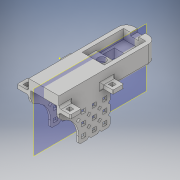
# Autodesk Inventor part: Milling Machine with light_sensor_mount
Saved by Autodesk Inventor 2017 SP1 (Build 210196100, 196)
## iProperties
Created: 2016-11-04
Part Number: Milling Machine with light_sensor_mount
Material: Generic
Document SubType Name: Modeling
Designer: rmainhar
Density: 1 g/cm^3
Appearance: Default
Author: rmainhar
Autodesk Inventor part; units mm, degrees
ref_plane "YZ Plane" through (0, 0, 0) normal (1, 0, 0) x (0, 1, 0)
ref_plane "XZ Plane" through (0, 0, 0) normal (0, 1, 0) x (-1, 0, 0)
ref_plane "XY Plane" through (0, 0, 0) normal (0, 0, 1) x (1, 0, 0)
sketch "Sketch1" plane through (0, 0, 0) normal (0, 1, 0) x (-1, 0, 0)
  line L0 (0, -12.7) -> (-63.5, -12.7)
  line L1 (-63.5, -12.7) -> (-63.5, 0)
  line L2 (-63.5, 0) -> (0, 0)
  line L3 (0, 0) -> (0, -12.7)
  line L4 (-3.9687, -7.9375) -> (-8.7313, -7.9375)
  line L5 (-8.7313, -7.9375) -> (-8.7312, -3.175)
  line L6 (-8.7312, -3.175) -> (-3.9687, -3.175)
  line L7 (-3.9687, -3.175) -> (-3.9687, -7.9375)
  line L8 (-54.7687, -3.175) -> (-54.7687, -7.9375)
  line L9 (-54.7687, -7.9375) -> (-59.5312, -7.9375)
  line L10 (-59.5312, -3.175) -> (-54.7687, -3.175)
  line L11 (-59.5312, -7.9375) -> (-59.5312, -3.175)
  point P0 (0, 0)
  dimension "d0" = 63.5
  dimension "d1" = 4.7625
  dimension "d2" = 4.7625
  dimension "d4" = 3.175
  dimension "d5" = 12.7
  dimension "d6" = 3.9688
  dimension "d9" = 50.8
  dimension "d14" = 3.9688
  constraints: 24 end point, 4 parallel, 3 horizontal, 2 perpendicular, 1 coincident, 8 other
  measures "d0" distance of L1.end L2.end
  measures "d1" distance of L5.end L6.end
  measures "d2" distance of L4.end L5.end
  measures "d4" distance between parallel lines of L2 L6
  measures "d5" distance of L2.end L0.start
  measures "d6" distance between parallel lines of L3 L7
  measures "d9" distance of L6.end L8.start
  measures "d14" distance between parallel lines of L1 L11
extrude "Extrusion1" add sketch "Sketch1" along normal blind 3.175
sketch "Sketch2" plane through (0, 0, 0) normal (0, -1, 0) x (1, 0, 0)
  line L0 (41.91, -43.3549) -> (21.8148, -43.3549)
  line L1 (21.8148, -43.3549) -> (21.8148, -12.7)
  line L2 (21.8148, -12.7) -> (41.91, -12.7)
  line L3 (41.91, -12.7) -> (41.91, -43.3549)
  line L4 (0, -12.7) -> (63.5, -12.7) projected
  line L5 (63.5, -12.7) -> (0, -12.7) projected
  line L6 (31.75, -12.7) -> (31.75, 0)
  line L7 (48.26, -49.7049) -> (15.4648, -49.7049)
  line L8 (15.4648, -49.7049) -> (15.4648, -6.35)
  line L9 (15.4648, -6.35) -> (48.26, -6.35)
  line L10 (48.26, -6.35) -> (48.26, -49.7049)
  point P0 (0, 0)
  dimension "d17" = 20.32
  dimension "d18" = 6.35
  dimension "d81" = 30.6549
  constraints: 18 end point, 4 parallel, 2 perpendicular, 1 horizontal, 1 midpoint, 1 point on line, 1 vertical, 3 other
  measures "d17" diameter of L3 L6
  measures "d18" distance between parallel lines of L10 L3
  measures "d81" distance between parallel lines of L0 L4
extrude "Extrusion2" add sketch "Sketch2" along normal blind 10.16 contours L3 L4 L10 L7 L8 L1 L0 | L2 L6 L9 L10 L4 | L4 L8 L9 L6 L2
sketch "Sketch3" plane through (63.5, 3.175, -12.7) normal (0, 0, -1) x (-1, 0, 0)
  line L0 (21.59, -13.335) -> (41.6852, -13.335) projected
  line L1 (41.6852, -13.335) -> (21.59, -13.335) projected
  line L2 (48.0352, -13.335) -> (15.24, -13.335) projected
  line L3 (15.24, -13.335) -> (48.0352, -13.335) projected
  line L4 (63.5, -3.175) -> (48.0352, -3.175) projected
  line L5 (63.5, -3.175) -> (63.5, 0) projected
  line L6 (0, 0) -> (63.5, 0) projected
  line L7 (0, -3.175) -> (0, 0) projected
  line L8 (15.24, -3.175) -> (0, -3.175) projected
  line L9 (21.59, -3.175) -> (15.24, -3.175) projected
  line L10 (21.59, -3.175) -> (21.59, -13.335) projected
  line L11 (41.6852, -13.335) -> (21.59, -13.335) projected
  line L12 (41.6852, -3.175) -> (41.6852, -13.335) projected
  line L13 (48.0352, -3.175) -> (41.6852, -3.175) projected
  line L14 (21.59, -3.175) -> (41.6852, -3.175)
  line L15 (41.6852, -3.175) -> (41.6852, -13.335)
  line L16 (41.6852, -13.335) -> (21.59, -13.335)
  line L17 (21.59, -13.335) -> (21.59, -3.175)
  constraints: 8 end point, 2 parallel, 1 horizontal, 1 perpendicular
extrude "Extrusion3" cut sketch "Sketch3" against normal blind 12.7 contours L10 L14 L12 L0
sketch "Sketch4" plane through (0, 0, 0) normal (0, 1, 0) x (1, 0, 0)
  line L0 (41.91, 12.7) -> (48.26, 12.7) projected
  line L1 (48.26, 12.7) -> (48.26, 49.7049) projected
  line L2 (48.26, 49.7049) -> (15.4648, 49.7049) projected
  line L3 (15.4648, 49.7049) -> (15.4648, 12.7) projected
  line L4 (21.8148, 12.7) -> (21.8148, 43.3549) projected
  line L5 (21.8148, 43.3549) -> (41.91, 43.3549) projected
  line L6 (41.91, 43.3549) -> (41.91, 12.7) projected
  line L7 (15.4648, 12.7) -> (21.8148, 12.7) projected
  point P0 (0, 0)
extrude "Extrusion4" add sketch "Sketch4" along normal up to surface (3.175 mm away)
sketch "Sketch5" plane through (41.91, 0, -12.7) normal (0, 0, -1) x (-1, 0, 0)
  line L0 (0, 3.175) -> (0, 0) projected
  line L1 (0, 0) -> (20.0952, 0) projected
  line L2 (20.0952, 0) -> (20.0952, 3.175) projected
  line L3 (0, 3.175) -> (20.0952, 3.175) projected
  point P0 (41.91, 0)
extrude "Extrusion5" cut sketch "Sketch5" against normal through all
sketch "Sketch6" plane through (41.91, 0, -6.35) normal (-1, 0, 0) x (0, 0, 1)
  line L0 (0, 0) -> (-6.35, 0) projected
  line L1 (0, 0) -> (0, -10.16) projected
  line L2 (-43.3549, -10.16) -> (0, -10.16) projected
  line L3 (-43.3549, 3.175) -> (-43.3549, -10.16) projected
  line L4 (-43.3549, 3.175) -> (-6.35, 3.175) projected
  line L5 (-6.35, 0) -> (-6.35, 3.175) projected
  line L6 (3.175, 0) -> (3.175, 3.175) projected
  line L7 (-6.35, 0) -> (6.35, 0) projected
  line L8 (-6.35, 0) -> (-6.35, 3.175) projected
  line L9 (6.35, 3.175) -> (-6.35, 3.175) projected
  line L10 (6.35, 0) -> (6.35, 3.175) projected
  line L11 (-43.3549, -10.16) -> (0, -10.16) projected
  arc A0 (0, -10.16) -> (6.35, 0) centre (-4.953, 0) ccw
  line L12 (0, 0) -> (0, -10.16) projected
  line L13 (0, -10.16) -> (0, 0)
  line L14 (6.35, 0) -> (0, 0) projected
  line L15 (0, 0) -> (6.35, 0)
  constraints: 4 end point, 2 point on circle, 1 centre point, 1 collinear, 1 perpendicular, 1 tangent
extrude "Extrusion6" add sketch "Sketch6" against normal up to surface (6.35 mm away) contours L7 A0 L1
sketch "Sketch17" plane through (0, 0, 0) normal (0, -1, 0) x (1, 0, 0)
  line L0 (21.8148, -6.35) -> (21.8148, 0) projected
  line L1 (21.8148, 0) -> (0, 0) projected
  line L2 (0, 0) -> (0, -12.7) projected
  line L3 (0, -12.7) -> (15.4648, -12.7) projected
  line L4 (15.4648, -12.7) -> (15.4648, -6.35) projected
  line L5 (15.4648, -6.35) -> (21.8148, -6.35) projected
  line L6 (8.7312, -3.175) -> (8.7313, -7.9375) projected
  line L7 (8.7313, -7.9375) -> (3.9687, -7.9375) projected
  line L8 (3.9687, -7.9375) -> (3.9687, -3.175) projected
  line L9 (3.9687, -3.175) -> (8.7312, -3.175) projected
  point P0 (0, 0)
sketch "Sketch7" plane through (0, -10.16, 0) normal (0, -1, 0) x (1, 0, 0)
  line L0 (48.26, 0) -> (48.26, -12.7) projected
  line L1 (48.26, -12.7) -> (63.5, -12.7) projected
  line L2 (63.5, -12.7) -> (63.5, 0) projected
  line L3 (63.5, 0) -> (48.26, 0) projected
  line L4 (54.7687, -7.9375) -> (54.7687, -3.175) projected
  line L5 (54.7687, -3.175) -> (59.5312, -3.175) projected
  line L6 (59.5312, -3.175) -> (59.5312, -7.9375) projected
  line L7 (59.5312, -7.9375) -> (54.7687, -7.9375) projected
  line L8 (41.91, -6.35) -> (41.91, -43.3549) projected
  line L9 (41.91, -43.3549) -> (21.8148, -43.3549) projected
  line L10 (21.8148, -43.3549) -> (21.8148, -6.35) projected
  line L11 (21.8148, -6.35) -> (15.4648, -6.35) projected
  line L12 (15.4648, -6.35) -> (15.4648, -49.7049) projected
  line L13 (15.4648, -49.7049) -> (48.26, -49.7049) projected
  line L14 (48.26, -49.7049) -> (48.26, -6.35) projected
  line L15 (48.26, -6.35) -> (41.91, -6.35) projected
  line L16 (41.91, -43.3549) -> (41.91, 0) projected
  line L17 (41.91, 0) -> (63.5, 0) projected
  line L18 (48.26, 0) -> (41.91, 0)
  line L19 (41.91, 0) -> (41.91, -12.7)
  arc A0 (46.814, 0) -> (41.91, -12.7) centre (60.8067, -12.7) ccw
  line L20 (41.91, -6.35) -> (41.91, -43.3549) projected
  point P0 (0, 0)
  constraints: 4 end point, 2 point on circle, 2 point on line, 1 centre point, 1 collinear, 1 perpendicular, 1 tangent
extrude "Extrusion8" cut sketch "Sketch7" against normal through all contours A0 L15 L16 L17 | A0 L8 L15
ref_plane "Work Plane1" through (31.8624, -10.16, -43.3549) normal (-1, 0, 0) x (0, 0, 1)
mirror "Mirror1" about plane through (31.8624, -10.16, -43.3549) normal (-1, 0, 0) of "Extrusion8", "Extrusion6"
fillet "Fillet10" radius 1.524 5 edges at (42.1867, -10.16, -9.4778) (41.91, -10.16, -28.0275) (21.5381, -10.16, -9.4778) (21.8148, -10.16, -28.0275) (31.8624, -10.16, -43.3549)
sketch "Sketch8" plane through (0, 3.175, 0) normal (0, 1, 0) x (1, 0, 0)
  point P0 (0, 0)
sketch "Sketch9" plane through (0, 3.175, 0) normal (0, 1, 0) x (1, 0, 0)
  line L0 (13.8138, 65.5799) -> (49.911, 65.5799)
  line L1 (49.911, 65.5799) -> (49.911, -57.15)
  line L2 (49.911, -57.15) -> (13.8138, -57.15)
  line L3 (13.8138, -57.15) -> (13.8138, 65.5799)
  line L4 (15.4648, 49.7049) -> (48.26, 49.7049) projected
  line L5 (15.4648, 12.7) -> (15.4648, 49.7049) projected
  line L6 (15.4648, 12.7) -> (0, 12.7) projected
  line L7 (0, 12.7) -> (0, 0) projected
  line L8 (0, 0) -> (16.9108, 0) projected
  arc A0 (16.9108, 0) -> (21.8148, 12.7) centre (2.9181, 12.7) ccw projected
  line L9 (21.8148, 43.3549) -> (21.8148, 12.7) projected
  line L10 (41.91, 43.3549) -> (21.8148, 43.3549) projected
  line L11 (41.91, 43.3549) -> (41.91, 12.7) projected
  arc A1 (41.91, 12.7) -> (46.814, 0) centre (60.8067, 12.7) ccw projected
  line L12 (46.814, 0) -> (63.5, 0) projected
  line L13 (63.5, 0) -> (63.5, 12.7) projected
  line L14 (63.5, 12.7) -> (48.26, 12.7) projected
  line L15 (48.26, 49.7049) -> (48.26, 12.7) projected
  line L16 (8.7313, 7.9375) -> (8.7312, 3.175) projected
  line L17 (8.7312, 3.175) -> (3.9687, 3.175) projected
  line L18 (3.9687, 3.175) -> (3.9687, 7.9375) projected
  line L19 (3.9687, 7.9375) -> (8.7313, 7.9375) projected
  line L20 (54.7687, 3.175) -> (54.7687, 7.9375) projected
  line L21 (54.7687, 7.9375) -> (59.5312, 7.9375) projected
  line L22 (59.5312, 7.9375) -> (59.5312, 3.175) projected
  line L23 (59.5312, 3.175) -> (54.7687, 3.175) projected
  point P0 (0, 0)
  dimension "d44" = 15.875
  dimension "d80" = 57.15
  constraints: 8 end point, 2 parallel, 1 horizontal, 1 perpendicular
  measures "d44" distance between parallel lines of L0 L4
  measures "d80" distance between parallel lines of L2 L12
extrude "Extrusion9" add sketch "Sketch9" along normal blind 12.7 contours L0 L1 L14 L15 L4 L5 L6 L3 | L6 L5 L4 L15 L14 L1 L12 A1 L11 L10 L9 A0 L8 L3 | L8 A0 L9 L10 L11 A1 L12 L1 L2 L3
sketch "Sketch10" plane through (0, 3.175, 0) normal (0, -1, 0) x (1, 0, 0)
  line L0 (46.814, 0) -> (49.911, 0) projected
  line L1 (49.911, 0) -> (49.911, 57.15) projected
  line L2 (49.911, 57.15) -> (13.8138, 57.15) projected
  line L3 (13.8138, 57.15) -> (13.8138, 0) projected
  line L4 (13.8138, 0) -> (16.9108, 0) projected
  arc A0 (21.8148, -12.7) -> (16.9108, 0) centre (2.9181, -12.7) ccw projected
  line L5 (21.8148, -43.3549) -> (21.8148, -12.7) projected
  line L6 (41.91, -43.3549) -> (21.8148, -43.3549) projected
  line L7 (41.91, -43.3549) -> (41.91, -12.7) projected
  arc A1 (46.814, 0) -> (41.91, -12.7) centre (60.8067, -12.7) ccw projected
  circle A2 centre (31.8624, -33.8299) radius 4.0047
  point P0 (0, 0)
  dimension "d49" = 9.525
  constraints: 1 centre point
  measures "d49" distance from line of L6 A2.centre
extrude "Extrusion10" cut sketch "Sketch10" against normal through all contours A2
sketch "Sketch11" plane through (0, 15.875, 0) normal (0, 1, 0) x (1, 0, 0)
  circle A0 centre (31.8624, 33.8299) radius 4.0047 projected
  line L0 (18.6544, 57.6297) -> (45.0704, 57.6297)
  line L1 (45.0704, 57.6297) -> (45.0704, 24.6097)
  line L2 (45.0704, 24.6097) -> (18.6544, 24.6097)
  line L3 (18.6544, 24.6097) -> (18.6544, 57.6297)
  point P0 (0, 0)
  dimension "d52" = 13.208
  dimension "d53" = 13.208
  dimension "d54" = 23.7998
  dimension "d55" = 33.02
  constraints: 8 end point, 2 parallel, 1 horizontal, 1 perpendicular
  measures "d52" distance from line of L1 A0.centre
  measures "d53" distance from line of L3 A0.centre
  measures "d54" distance from line of L0 A0.centre
  measures "d55" distance between parallel lines of L2 L0
extrude "Extrusion11" cut sketch "Sketch11" against normal up to surface (12.7 mm away)
sketch "Sketch12" plane through (0, 15.875, 0) normal (0, 1, 0) x (1, 0, 0)
  line L0 (45.0704, 24.6097) -> (18.6544, 24.6097) projected
  line L1 (45.0704, 24.6097) -> (18.6544, 24.6097)
  line L2 (18.6544, 24.6097) -> (18.6544, 8.0997)
  line L3 (18.6544, 8.0997) -> (45.0704, 8.0997)
  line L4 (45.0704, 8.0997) -> (45.0704, 24.6097)
  point P0 (0, 0)
  dimension "d58" = 16.51
  constraints: 8 end point, 2 parallel, 1 horizontal, 1 perpendicular
  measures "d58" distance of L2.end L1.end
extrude "Extrusion12" cut sketch "Sketch12" against normal blind 7.62
sketch "Sketch14" plane through (0, 15.875, 0) normal (0, 1, 0) x (1, 0, 0)
  line L0 (18.6544, 57.6297) -> (45.0704, 57.6297) projected
  line L1 (36.6249, 57.6297) -> (27.0999, 57.6297)
  line L2 (27.0999, 57.6297) -> (27.0999, 66.8243)
  line L3 (27.0999, 66.8243) -> (36.6249, 66.8243)
  line L4 (36.6249, 66.8243) -> (36.6249, 57.6297)
  line L5 (31.8624, -81.9449) -> (31.8624, 91.6192) projected
  line L6 (49.911, 65.5799) -> (13.8138, 65.5799) projected
  point P0 (0, 0)
  dimension "d64" = 4.7625
  dimension "d65" = 4.7625
  constraints: 8 end point, 2 parallel, 1 horizontal, 1 perpendicular, 1 point on line
  measures "d64" distance between parallel lines of L2 L5
  measures "d65" distance between parallel lines of L4 L5
extrude "Extrusion14" cut sketch "Sketch14" against normal blind 5.08
sketch "Sketch15" plane through (18.6544, 3.175, -57.6297) normal (1, 0, 0) x (0, 0, -1)
  line L0 (-33.02, 0) -> (-7.9248, 0) projected
  line L1 (-33.02, 5.08) -> (-33.02, 0) projected
  arc A0 (-33.02, 1.5875) -> (-31.4325, 0) centre (-31.4325, 1.5875) ccw
  line L2 (-33.02, 0) -> (-31.4325, 0)
  line L3 (-33.02, 0) -> (-33.02, 1.5875)
  point P0 (-57.6297, -3.175)
  point P1 (0, 0)
  dimension "d68" = 3.175
  constraints: 4 end point, 2 point on circle, 2 point on line, 2 tangent, 1 centre point
  measures "d68" diameter of A0
extrude "Extrusion15" add sketch "Sketch15" along normal up to surface (26.416 mm away)
fillet "Fillet13" radius 9.525 2 edges at (49.911, 9.525, -65.5799) (13.8138, 9.525, -65.5799)
fillet "Fillet17" radius 0.762 2 edges at (48.3625, 3.175, 0) (15.3623, 3.175, 0)
sketch "Sketch16" plane through (0, 8.255, 0) normal (0, 1, 0) x (1, 0, 0)
  line L0 (31.8624, -81.696) -> (31.8624, 90.1259)
  circle A0 centre (31.8624, 18.2597) radius 4.7625
  line L1 (18.6544, 24.6097) -> (45.0704, 24.6097)
  line L2 (8.7312, 3.175) -> (8.7313, 7.9375)
  line L3 (8.7313, 7.9375) -> (3.9687, 7.9375)
  line L4 (3.9687, 7.9375) -> (3.9687, 3.175)
  line L5 (3.9687, 3.175) -> (8.7312, 3.175)
  line L6 (0, 1.524) -> (12.2898, 1.524)
  line L7 (0, 1.524) -> (0, 12.7)
  line L8 (0, 12.7) -> (12.2898, 12.7)
  line L9 (12.2898, 1.524) -> (12.2898, 12.7)
  point P0 (0, 0)
  point P1 (6.35, 5.5563)
  dimension "d76" = 9.525
  dimension "d77" = 6.35
  dimension "d82" = 12.7035
  constraints: 20 end point, 1 centre point, 1 point on line
  measures "d76" diameter of A0
  measures "d77" distance from line of L1 A0.centre
  measures "d82" vertical distance of point (6.35, 5.556) A0.centre
extrude "Extrusion16" cut sketch "Sketch16" against normal through all contours A0 L0 | L0 A0
sketch "Sketch13" plane through (0, -10.16, 0) normal (0, -1, 0) x (1, 0, 0)
  line L0 (67.084, -58.3432) -> (-5.543, -58.3432)
  line L1 (-5.543, -58.3432) -> (-5.543, 19.1161)
  line L2 (-5.543, 19.1161) -> (67.084, 19.1161)
  line L3 (67.084, 19.1161) -> (67.084, -58.3432)
  point P0 (0, 0)
  constraints: 8 end point, 2 parallel, 1 horizontal, 1 perpendicular
extrude "Extrusion13" cut sketch "Sketch13" against normal blind 2.54
sketch "Sketch18" plane through (0, 3.175, 0) normal (0, -1, 0) x (1, 0, 0)
  line L0 (16.176, 50.9532) -> (0, 50.9532)
  line L1 (0, 50.9532) -> (0, 38.2532)
  line L2 (0, 38.2532) -> (16.176, 38.2532)
  line L3 (16.176, 38.2532) -> (16.176, 50.9532)
  line L4 (8.7313, 47.7782) -> (8.7313, 43.0157)
  line L5 (8.7313, 43.0157) -> (3.9688, 43.0157)
  line L6 (3.9688, 43.0157) -> (3.9688, 47.7782)
  line L7 (3.9688, 47.7782) -> (8.7313, 47.7782)
  line L8 (13.8138, 57.15) -> (13.8138, 0.762)
  circle A0 centre (31.8624, -18.2597) radius 4.7625
  arc A1 (21.8148, -12.7) -> (16.1794, 0.762) centre (2.9181, -12.7) ccw
  line L9 (21.8148, -26.1972) -> (21.8148, -12.7)
  line L10 (21.8148, -26.1972) -> (41.91, -26.1972)
  line L11 (41.91, -26.1972) -> (41.91, -12.7)
  arc A2 (47.5455, 0.762) -> (41.91, -12.7) centre (60.8067, -12.7) ccw
  line L12 (49.911, 0.762) -> (47.5455, 0.762)
  line L13 (49.911, 0.762) -> (49.911, 57.15)
  line L14 (49.911, 57.15) -> (13.8138, 57.15)
  line L15 (13.8138, 57.15) -> (13.8138, 0.762)
  line L16 (16.1794, 0.762) -> (13.8138, 0.762)
  line L17 (0, -1.524) -> (0, 0)
  point P0 (-3.9646, 51.0441)
  point P1 (6.35, -5.403)
  point P2 (6.35, 45.397)
  dimension "d83" = 4.7625
  dimension "d84" = 4.7625
  dimension "d85" = 3.9688
  dimension "d86" = 3.175
  dimension "d87" = 4.7625
  dimension "d89" = 0
  dimension "d92" = 50.8
  dimension "d93" = 2.3813
  dimension "d94" = 2.3813
  dimension "d102" = 2.3622
  constraints: 36 end point, 4 point on circle, 3 centre point, 3 perpendicular, 1 other
  measures "d83" distance of L6.end L4.start
  measures "d84" distance of L4.start L4.end
  measures "d85" distance between parallel lines of L1 L6
  measures "d86" distance between parallel lines of L0 L7
  measures "d87" distance between parallel lines of L2 L5
  measures "d89" distance between parallel lines of L17 L1
  measures "d92" distance of point (6.35, -5.403) point (6.35, 45.397)
  measures "d93" distance from line of L7 point (6.35, 45.397)
  measures "d94" distance from line of L6 point (6.35, 45.397)
  measures "d102" distance between parallel lines of L3 L8
extrude "Extrusion17" add sketch "Sketch18" along normal blind 5.08 contours L3 L2 L8 L0 | L8 L2 L1 L0
ref_plane "Work Plane4" through (16.3538, 3.175, 57.15) normal (-1, 0, 0) x (0, 0, 1)
sketch "Sketch20" plane through (16.3538, 3.175, 57.15) normal (-1, 0, 0) x (0, 0, 1)
  line L0 (-65.0875, -25.4) -> (-67.3685, -23.119)
  line L1 (-65.0875, -25.4) -> (-56.9495, -25.4)
  line L2 (-54.6685, -23.119) -> (-56.9495, -25.4)
  line L3 (-52.3875, -25.4) -> (-54.6685, -23.119)
  line L4 (-52.3875, -25.4) -> (-44.2495, -25.4)
  line L5 (-41.9685, -23.119) -> (-44.2495, -25.4)
  line L6 (-39.6875, -25.4) -> (-41.9685, -23.119)
  line L7 (-39.6875, -25.4) -> (-31.5495, -25.4)
  line L8 (-29.2685, -23.119) -> (-31.5495, -25.4)
  line L9 (-26.9875, -25.4) -> (-29.2685, -23.119)
  line L10 (-26.9875, -25.4) -> (-18.8495, -25.4)
  line L11 (-16.5685, -23.119) -> (-18.8495, -25.4)
  line L12 (-14.2875, -25.4) -> (-16.5685, -23.119)
  line L13 (-14.2875, -25.4) -> (-6.1495, -25.4)
  line L14 (-3.8685, -23.119) -> (-6.1495, -25.4)
  line L15 (-65.0875, -12.7) -> (-67.3685, -10.419)
  line L16 (-67.3685, -14.981) -> (-65.0875, -12.7)
  line L17 (-41.9685, -10.419) -> (-44.2495, -12.7)
  line L18 (-39.6875, -12.7) -> (-41.9685, -10.419)
  line L19 (-41.9685, -14.981) -> (-39.6875, -12.7)
  line L20 (-44.2495, -12.7) -> (-41.9685, -14.981)
  line L21 (-16.5685, -10.419) -> (-18.8495, -12.7)
  line L22 (-14.2875, -12.7) -> (-16.5685, -10.419)
  line L23 (-16.5685, -14.981) -> (-14.2875, -12.7)
  line L24 (-18.8495, -12.7) -> (-16.5685, -14.981)
  line L25 (-54.6685, -2.281) -> (-52.3875, 0)
  line L26 (-56.9495, 0) -> (-54.6685, -2.281)
  line L27 (-29.2685, -2.281) -> (-26.9875, 0)
  line L28 (-31.5495, 0) -> (-29.2685, -2.281)
  line L29 (-6.1495, 0) -> (-3.8685, -2.281)
  line L30 (-12.5299, -8.6614) -> (-7.9071, -8.6614)
  line L31 (-12.5299, -4.0386) -> (-12.5299, -8.6614)
  line L32 (-7.9071, -4.0386) -> (-12.5299, -4.0386)
  line L33 (-7.9071, -8.6614) -> (-7.9071, -4.0386)
  line L34 (-25.2299, -8.6614) -> (-20.6071, -8.6614)
  line L35 (-25.2299, -4.0386) -> (-25.2299, -8.6614)
  line L36 (-20.6071, -4.0386) -> (-25.2299, -4.0386)
  line L37 (-20.6071, -8.6614) -> (-20.6071, -4.0386)
  line L38 (-37.9299, -8.6614) -> (-33.3071, -8.6614)
  line L39 (-37.9299, -4.0386) -> (-37.9299, -8.6614)
  line L40 (-33.3071, -4.0386) -> (-37.9299, -4.0386)
  line L41 (-33.3071, -8.6614) -> (-33.3071, -4.0386)
  line L42 (-50.6299, -8.6614) -> (-46.0071, -8.6614)
  line L43 (-50.6299, -4.0386) -> (-50.6299, -8.6614)
  line L44 (-46.0071, -4.0386) -> (-50.6299, -4.0386)
  line L45 (-46.0071, -8.6614) -> (-46.0071, -4.0386)
  line L46 (-63.3299, -8.6614) -> (-58.7071, -8.6614)
  line L47 (-63.3299, -4.0386) -> (-63.3299, -8.6614)
  line L48 (-58.7071, -4.0386) -> (-63.3299, -4.0386)
  line L49 (-58.7071, -8.6614) -> (-58.7071, -4.0386)
  line L50 (-12.5299, -21.3614) -> (-7.9071, -21.3614)
  line L51 (-12.5299, -16.7386) -> (-12.5299, -21.3614)
  line L52 (-7.9071, -16.7386) -> (-12.5299, -16.7386)
  line L53 (-7.9071, -21.3614) -> (-7.9071, -16.7386)
  line L54 (-25.2299, -21.3614) -> (-20.6071, -21.3614)
  line L55 (-25.2299, -16.7386) -> (-25.2299, -21.3614)
  line L56 (-20.6071, -16.7386) -> (-25.2299, -16.7386)
  line L57 (-20.6071, -21.3614) -> (-20.6071, -16.7386)
  line L58 (-37.9299, -21.3614) -> (-33.3071, -21.3614)
  line L59 (-37.9299, -16.7386) -> (-37.9299, -21.3614)
  line L60 (-33.3071, -16.7386) -> (-37.9299, -16.7386)
  line L61 (-33.3071, -21.3614) -> (-33.3071, -16.7386)
  line L62 (-50.6299, -21.3614) -> (-46.0071, -21.3614)
  line L63 (-50.6299, -16.7386) -> (-50.6299, -21.3614)
  line L64 (-46.0071, -16.7386) -> (-50.6299, -16.7386)
  line L65 (-46.0071, -21.3614) -> (-46.0071, -16.7386)
  line L66 (-63.3299, -21.3614) -> (-58.7071, -21.3614)
  line L67 (-63.3299, -16.7386) -> (-63.3299, -21.3614)
  line L68 (-58.7071, -16.7386) -> (-63.3299, -16.7386)
  line L69 (-58.7071, -21.3614) -> (-58.7071, -16.7386)
  line L70 (-16.5685, -2.281) -> (-14.2875, 0)
  line L71 (-18.8495, 0) -> (-16.5685, -2.281)
  line L72 (-41.9685, -2.281) -> (-39.6875, 0)
  line L73 (-44.2495, 0) -> (-41.9685, -2.281)
  line L74 (-67.3685, -2.281) -> (-65.0875, 0)
  line L75 (-3.8685, -10.419) -> (-6.1495, -12.7)
  line L76 (-6.1495, -12.7) -> (-3.8685, -14.981)
  line L77 (-29.2685, -10.419) -> (-31.5495, -12.7)
  line L78 (-26.9875, -12.7) -> (-29.2685, -10.419)
  line L79 (-29.2685, -14.981) -> (-26.9875, -12.7)
  line L80 (-31.5495, -12.7) -> (-29.2685, -14.981)
  line L81 (-54.6685, -10.419) -> (-56.9495, -12.7)
  line L82 (-52.3875, -12.7) -> (-54.6685, -10.419)
  line L83 (-54.6685, -14.981) -> (-52.3875, -12.7)
  line L84 (-56.9495, -12.7) -> (-54.6685, -14.981)
  line L85 (-65.0875, 0) -> (-56.9495, 0)
  line L86 (-52.3875, 0) -> (-44.2495, 0)
  line L87 (-39.6875, 0) -> (-31.5495, 0)
  line L88 (-26.9875, 0) -> (-18.8495, 0)
  line L89 (-14.2875, 0) -> (-6.1495, 0)
  line L90 (-67.3685, -2.281) -> (-67.3685, -10.419)
  line L91 (-67.3685, -14.981) -> (-67.3685, -23.119)
  line L92 (-3.8685, -23.119) -> (-3.8685, -14.981)
  line L93 (-3.8685, -10.419) -> (-3.8685, -2.281)
  line L94 (-65.0875, -3.175) -> (-65.0875, 0) projected
  line L95 (-56.388, 0) -> (-69.85, 0) projected
  line L96 (-14.2875, -38.1) -> (-16.5685, -35.819)
  line L97 (-3.8685, -35.819) -> (-6.1495, -38.1)
  line L98 (-12.5299, -34.0614) -> (-7.9071, -34.0614)
  line L99 (-16.5685, -35.819) -> (-18.8495, -38.1)
  line L100 (-7.9071, -34.0614) -> (-7.9071, -29.4386)
  line L101 (-12.5299, -29.4386) -> (-12.5299, -34.0614)
  line L102 (-7.9071, -29.4386) -> (-12.5299, -29.4386)
  line L103 (-3.8685, -35.819) -> (-3.8685, -27.681)
  line L104 (-6.1495, -25.4) -> (-3.8685, -27.681)
  line L105 (-14.2875, -25.4) -> (-6.1495, -25.4)
  line L106 (-16.5685, -27.681) -> (-14.2875, -25.4)
  line L107 (-25.2299, -34.0614) -> (-20.6071, -34.0614)
  line L108 (-20.6071, -34.0614) -> (-20.6071, -29.4386)
  line L109 (-18.8495, -25.4) -> (-16.5685, -27.681)
  line L110 (-25.2299, -29.4386) -> (-25.2299, -34.0614)
  line L111 (-20.6071, -29.4386) -> (-25.2299, -29.4386)
  line L112 (-26.9875, -25.4) -> (-18.8495, -25.4)
  line L113 (-46.0071, -46.7614) -> (-46.0071, -42.1386)
  line L114 (-26.9875, -50.8) -> (-29.2685, -48.519)
  line L115 (-29.2685, -48.519) -> (-31.5495, -50.8)
  line L116 (-33.3071, -42.1386) -> (-37.9299, -42.1386)
  line L117 (-33.3071, -46.7614) -> (-33.3071, -42.1386)
  line L118 (-37.9299, -42.1386) -> (-37.9299, -46.7614)
  line L119 (-37.9299, -46.7614) -> (-33.3071, -46.7614)
  line L120 (-39.6875, -50.8) -> (-31.5495, -50.8)
  line L121 (-41.9685, -48.519) -> (-44.2495, -50.8)
  line L122 (-39.6875, -50.8) -> (-41.9685, -48.519)
  line L123 (-50.6299, -42.1386) -> (-50.6299, -46.7614)
  line L124 (-52.3875, -50.8) -> (-44.2495, -50.8)
  line L125 (-50.6299, -46.7614) -> (-46.0071, -46.7614)
  line L126 (-46.0071, -42.1386) -> (-50.6299, -42.1386)
  line L127 (-44.2495, -25.4) -> (-41.9685, -27.681)
  line L128 (-46.0071, -34.0614) -> (-46.0071, -29.4386)
  line L129 (-50.6299, -34.0614) -> (-46.0071, -34.0614)
  line L130 (-50.6299, -29.4386) -> (-50.6299, -34.0614)
  line L131 (-52.3875, -25.4) -> (-44.2495, -25.4)
  line L132 (-54.6685, -27.681) -> (-52.3875, -25.4)
  line L133 (-46.0071, -29.4386) -> (-50.6299, -29.4386)
  line L134 (-67.3685, -27.681) -> (-65.0875, -25.4)
  line L135 (-63.3299, -34.0614) -> (-58.7071, -34.0614)
  line L136 (-63.3299, -29.4386) -> (-63.3299, -34.0614)
  line L137 (-58.7071, -34.0614) -> (-58.7071, -29.4386)
  line L138 (-58.7071, -29.4386) -> (-63.3299, -29.4386)
  line L139 (-65.0875, -25.4) -> (-56.9495, -25.4)
  line L140 (-56.9495, -25.4) -> (-54.6685, -27.681)
  line L141 (-29.2685, -35.819) -> (-31.5495, -38.1)
  line L142 (-39.6875, -38.1) -> (-41.9685, -35.819)
  line L143 (-41.9685, -35.819) -> (-44.2495, -38.1)
  line L144 (-44.2495, -38.1) -> (-41.9685, -40.381)
  line L145 (-41.9685, -40.381) -> (-39.6875, -38.1)
  line L146 (-31.5495, -38.1) -> (-29.2685, -40.381)
  line L147 (-29.2685, -40.381) -> (-26.9875, -38.1)
  line L148 (-37.9299, -34.0614) -> (-33.3071, -34.0614)
  line L149 (-37.9299, -29.4386) -> (-37.9299, -34.0614)
  line L150 (-26.9875, -38.1) -> (-29.2685, -35.819)
  line L151 (-33.3071, -29.4386) -> (-37.9299, -29.4386)
  line L152 (-33.3071, -34.0614) -> (-33.3071, -29.4386)
  line L153 (-41.9685, -27.681) -> (-39.6875, -25.4)
  line L154 (-39.6875, -25.4) -> (-31.5495, -25.4)
  line L155 (-31.5495, -25.4) -> (-29.2685, -27.681)
  line L156 (-29.2685, -27.681) -> (-26.9875, -25.4)
  line L157 (-65.0875, -38.1) -> (-67.3685, -35.819)
  line L158 (-54.6685, -35.819) -> (-56.9495, -38.1)
  line L159 (-52.3875, -38.1) -> (-54.6685, -35.819)
  line L160 (-56.9495, -38.1) -> (-54.6685, -40.381)
  line L161 (-54.6685, -40.381) -> (-52.3875, -38.1)
  line L162 (-67.3685, -40.381) -> (-65.0875, -38.1)
  line L163 (-58.7071, -42.1386) -> (-63.3299, -42.1386)
  line L164 (-58.7071, -46.7614) -> (-58.7071, -42.1386)
  line L165 (-63.3299, -46.7614) -> (-58.7071, -46.7614)
  line L166 (-63.3299, -42.1386) -> (-63.3299, -46.7614)
  line L167 (-52.3875, -50.8) -> (-54.6685, -48.519)
  line L168 (-54.6685, -48.519) -> (-56.9495, -50.8)
  line L169 (-65.0875, -50.8) -> (-56.9495, -50.8)
  line L170 (-67.3685, -40.381) -> (-67.3685, -48.519)
  line L171 (-65.0875, -50.8) -> (-67.3685, -48.519)
  line L172 (-20.6071, -42.1386) -> (-25.2299, -42.1386)
  line L173 (-20.6071, -46.7614) -> (-20.6071, -42.1386)
  line L174 (-25.2299, -42.1386) -> (-25.2299, -46.7614)
  line L175 (-25.2299, -46.7614) -> (-20.6071, -46.7614)
  line L176 (-26.9875, -50.8) -> (-18.8495, -50.8)
  line L177 (-6.1495, -38.1) -> (-3.8685, -40.381)
  line L178 (-18.8495, -38.1) -> (-16.5685, -40.381)
  line L179 (-16.5685, -40.381) -> (-14.2875, -38.1)
  line L180 (-7.9071, -42.1386) -> (-12.5299, -42.1386)
  line L181 (-7.9071, -46.7614) -> (-7.9071, -42.1386)
  line L182 (-12.5299, -42.1386) -> (-12.5299, -46.7614)
  line L183 (-3.8685, -48.519) -> (-3.8685, -40.381)
  line L184 (-12.5299, -46.7614) -> (-7.9071, -46.7614)
  line L185 (-16.5685, -48.519) -> (-18.8495, -50.8)
  line L186 (-14.2875, -50.8) -> (-16.5685, -48.519)
  line L187 (-14.2875, -50.8) -> (-6.1495, -50.8)
  line L188 (-3.8685, -48.519) -> (-6.1495, -50.8)
  line L189 (-67.3685, -27.681) -> (-67.3685, -35.819)
  dimension "d118" = 25.4
  constraints: 376 end point, 2 collinear, 2 vertical, 187 other
  measures "d118" distance of L22.end L96.end
extrude "Extrusion21" add sketch "Sketch20" along normal up to surface (2.54 mm away) contours L0 L91 L16 L15 L90 L74 L85 L26 L25 L86 L73 L72 L87 L28 L27 L88 L71 L70 L89 L29 L93 L75 L76 L92 L14 L13 L12 L11 L10 L9 L8 L7 L6 L5 L4 L3 L2 L1 | L1 L140 L132 L4 L127 L153 L7 L155 L156 L10 L109 L106 L13 L104 L103 L97 L177 L183 L188 L187 L186 L185 L176 L114 L115 L120 L122 L121 L124 L167 L168 L169 L171 L170 L162 L157 L189 L134
sketch "Sketch25" plane through (16.3538, 3.175, 57.15) normal (1, 0, 0) x (0, 0, -1)
  line L0 (3.8685, -2.281) -> (3.8685, -10.419) projected
  line L1 (18.8968, 0) -> (6.1968, 0) projected
  line L2 (67.3685, -14.981) -> (65.0875, -12.7) projected
  line L3 (0, 0) -> (6.1495, 0) projected
  line L4 (67.3685, -14.981) -> (3.8685, -14.981)
  line L5 (3.8685, -14.981) -> (3.8685, 0)
  line L6 (3.8685, 0) -> (67.3685, 0)
  line L7 (67.3685, 0) -> (67.3685, -14.981)
  point P0 (67.3685, -23.119)
  constraints: 8 end point, 2 parallel, 1 horizontal, 1 perpendicular, 1 point on line
extrude "Extrusion22" add sketch "Sketch25" against normal up to surface (2.54 mm away)
ref_plane "Work Plane5" through (31.8624, 3.175, 57.15) normal (-1, 0, 0) x (0, 0, 1)
mirror "Mirror2" about plane through (31.8624, 3.175, 57.15) normal (-1, 0, 0) of "Extrusion17"
mirror "Mirror3" about plane through (31.8624, 3.175, 57.15) normal (-1, 0, 0) of "Extrusion21", "Extrusion22"
sketch "Sketch35" plane through (0, 15.875, 0) normal (0, 1, 0) x (1, 0, 0)
  line L0 (47.371, -51.0005) -> (49.911, -51.0005) projected
  line L1 (47.371, -53.2815) -> (49.911, -53.2815) projected
  line L2 (13.8138, 56.0549) -> (13.8138, -57.15) projected
  line L3 (49.911, -57.15) -> (49.911, 56.0549) projected
  line L4 (51.435, -50.9532) -> (8.9069, -50.9532)
  line L5 (8.9069, -50.9532) -> (8.9069, -59.5888)
  line L6 (8.9069, -59.5888) -> (51.435, -59.5888)
  line L7 (51.435, -59.5888) -> (51.435, -50.9532)
  point P0 (0, 0)
  constraints: 8 end point, 2 parallel, 1 perpendicular
extrude "Extrusion29" cut sketch "Sketch35" against normal through all
sketch "Sketch37" plane through (0, 15.875, 0) normal (0, 1, 0) x (1, 0, 0)
  line L0 (13.8138, -50.9532) -> (49.911, -50.9532) projected
  line L1 (49.911, -50.9532) -> (49.911, 56.0549) projected
  arc A0 (49.911, 56.0549) -> (40.386, 65.5799) centre (40.386, 56.0549) ccw projected
  line L2 (40.386, 65.5799) -> (36.6249, 65.5799) projected
  line L3 (36.6249, 65.5799) -> (36.6249, 57.6297) projected
  line L4 (36.6249, 57.6297) -> (45.0704, 57.6297) projected
  line L5 (45.0704, 57.6297) -> (45.0704, 8.0997) projected
  line L6 (45.0704, 8.0997) -> (18.6544, 8.0997) projected
  line L7 (18.6544, 8.0997) -> (18.6544, 57.6297) projected
  line L8 (18.6544, 57.6297) -> (27.0999, 57.6297) projected
  line L9 (27.0999, 57.6297) -> (27.0999, 65.5799) projected
  line L10 (27.0999, 65.5799) -> (23.3388, 65.5799) projected
  arc A1 (23.3388, 65.5799) -> (13.8138, 56.0549) centre (23.3388, 56.0549) ccw projected
  line L11 (13.8138, 56.0549) -> (13.8138, -50.9532) projected
  point P0 (0, 0)
extrude "Extrusion30" cut sketch "Sketch37" against normal blind 1.27
sketch "Sketch39" plane through (0, 3.175, 0) normal (0, 1, 0) x (1, 0, 0)
  line L0 (13.8138, 0) -> (13.8138, 12.7) projected
  line L1 (13.8138, 12.7) -> (0, 12.7) projected
  line L2 (0, 12.7) -> (0, 0) projected
  line L3 (0, 0) -> (13.8138, 0) projected
  line L4 (8.7313, 7.9375) -> (8.7312, 3.175) projected
  line L5 (8.7312, 3.175) -> (3.9687, 3.175) projected
  line L6 (3.9687, 3.175) -> (3.9687, 7.9375) projected
  line L7 (3.9687, 7.9375) -> (8.7313, 7.9375) projected
  line L8 (54.7687, 3.175) -> (54.7687, 7.9375) projected
  line L9 (54.7687, 7.9375) -> (59.5312, 7.9375) projected
  line L10 (59.5312, 7.9375) -> (59.5312, 3.175) projected
  line L11 (59.5312, 3.175) -> (54.7687, 3.175) projected
  line L12 (49.911, 12.7) -> (49.911, 0) projected
  line L13 (49.911, 0) -> (63.5, 0) projected
  line L14 (63.5, 0) -> (63.5, 12.7) projected
  line L15 (63.5, 12.7) -> (49.911, 12.7) projected
  line L16 (63.7248, -50.9532) -> (63.7248, -38.2532) projected
  line L17 (63.7248, -38.2532) -> (49.911, -38.2532) projected
  line L18 (59.7561, -43.0157) -> (54.9936, -43.0157) projected
  line L19 (59.7561, -47.7782) -> (59.7561, -43.0157) projected
  line L20 (54.9936, -47.7782) -> (59.7561, -47.7782) projected
  line L21 (54.9936, -43.0157) -> (54.9936, -47.7782) projected
  line L22 (0, -38.2532) -> (13.8138, -38.2532) projected
  line L23 (0, -50.9532) -> (0, -38.2532) projected
  line L24 (13.8138, -50.9532) -> (0, -50.9532) projected
  line L25 (3.9688, -43.0157) -> (8.7313, -43.0157) projected
  line L26 (8.7313, -43.0157) -> (8.7313, -47.7782) projected
  line L27 (8.7313, -47.7782) -> (3.9688, -47.7782) projected
  line L28 (3.9688, -47.7782) -> (3.9688, -43.0157) projected
  line L29 (13.8138, -50.9532) -> (13.8138, -38.2532) projected
  line L30 (49.911, -38.2532) -> (49.911, -50.9532) projected
  line L31 (49.911, -50.9532) -> (63.7248, -50.9532) projected
  point P0 (0, 0)
extrude "Extrusion31" cut sketch "Sketch39" against normal blind 1.27
sketch "Sketch40" plane through (0, 0, 0) normal (0, -1, 0) x (1, 0, 0)
  line L0 (15.4648, -10.2185) -> (13.8138, -10.2185) projected
  line L1 (13.8138, -10.2185) -> (13.8138, 0) projected
  line L2 (13.8138, 0) -> (0, 0) projected
  line L3 (0, 0) -> (0, -12.7) projected
  line L4 (0, -12.7) -> (15.4648, -12.7) projected
  line L5 (15.4648, -12.7) -> (15.4648, -10.2185) projected
  line L6 (8.7312, -3.175) -> (8.7313, -7.9375) projected
  line L7 (8.7313, -7.9375) -> (3.9687, -7.9375) projected
  line L8 (3.9687, -7.9375) -> (3.9687, -3.175) projected
  line L9 (3.9687, -3.175) -> (8.7312, -3.175) projected
  line L10 (49.911, -10.2185) -> (48.26, -10.2185) projected
  line L11 (48.26, -10.2185) -> (48.26, -12.7) projected
  line L12 (48.26, -12.7) -> (63.5, -12.7) projected
  line L13 (63.5, -12.7) -> (63.5, 0) projected
  line L14 (63.5, 0) -> (49.911, 0) projected
  line L15 (49.911, 0) -> (49.911, -10.2185) projected
  line L16 (54.7687, -7.9375) -> (54.7687, -3.175) projected
  line L17 (54.7687, -3.175) -> (59.5312, -3.175) projected
  line L18 (59.5312, -3.175) -> (59.5312, -7.9375) projected
  line L19 (59.5312, -7.9375) -> (54.7687, -7.9375) projected
  line L20 (49.911, 50.9532) -> (49.911, 38.2532) projected
  line L21 (63.7248, 38.2532) -> (49.911, 38.2532) projected
  line L22 (63.7248, 50.9532) -> (63.7248, 38.2532) projected
  line L23 (49.911, 50.9532) -> (63.7248, 50.9532) projected
  line L24 (54.9936, 43.0157) -> (59.7561, 43.0157) projected
  line L25 (54.9936, 47.7782) -> (54.9936, 43.0157) projected
  line L26 (59.7561, 47.7782) -> (54.9936, 47.7782) projected
  line L27 (59.7561, 43.0157) -> (59.7561, 47.7782) projected
  line L28 (13.8138, 38.2532) -> (13.8138, 50.9532) projected
  line L29 (13.8138, 50.9532) -> (0, 50.9532) projected
  line L30 (0, 50.9532) -> (0, 38.2532) projected
  line L31 (0, 38.2532) -> (13.8138, 38.2532) projected
  line L32 (8.7313, 43.0157) -> (3.9688, 43.0157) projected
  line L33 (3.9688, 43.0157) -> (3.9688, 47.7782) projected
  line L34 (3.9688, 47.7782) -> (8.7313, 47.7782) projected
  line L35 (8.7313, 47.7782) -> (8.7313, 43.0157) projected
  point P0 (0, 0)
extrude "Extrusion32" add sketch "Sketch40" along normal blind 2.54
sketch "Sketch43" plane through (0, 3.175, 0) normal (0, -1, 0) x (1, 0, 0)
  arc A0 (13.8138, -56.0549) -> (23.3388, -65.5799) centre (23.3388, -56.0549) ccw projected
  line L0 (23.3388, -65.5799) -> (40.386, -65.5799) projected
  arc A1 (40.386, -65.5799) -> (49.911, -56.0549) centre (40.386, -56.0549) ccw projected
  line L1 (49.911, -56.0549) -> (49.911, -12.7) projected
  line L2 (49.911, -12.7) -> (48.26, -12.7) projected
  line L3 (48.26, -49.7049) -> (48.26, -12.7) projected
  line L4 (45.0704, -49.7049) -> (48.26, -49.7049) projected
  line L5 (45.0704, -49.7049) -> (45.0704, -57.6297) projected
  line L6 (45.0704, -57.6297) -> (18.6544, -57.6297) projected
  line L7 (18.6544, -57.6297) -> (18.6544, -49.7049) projected
  line L8 (15.4648, -49.7049) -> (18.6544, -49.7049) projected
  line L9 (15.4648, -12.7) -> (15.4648, -49.7049) projected
  line L10 (15.4648, -12.7) -> (13.8138, -12.7) projected
  line L11 (13.8138, -12.7) -> (13.8138, -56.0549) projected
  line L12 (18.6544, -57.6297) -> (18.6544, -49.7049) projected
  line L13 (18.6544, -57.6297) -> (45.0704, -57.6297)
  line L14 (45.0704, -57.6297) -> (45.0704, -49.7049)
  line L15 (45.0704, -49.7049) -> (18.6544, -49.7049)
  line L16 (18.6544, -49.7049) -> (18.6544, -57.6297)
  line L17 (13.8138, -7.9375) -> (13.8138, -10.2185) projected
  line L18 (16.3538, -10.2185) -> (13.8138, -10.2185) projected
  line L19 (16.3538, -7.9375) -> (16.3538, -10.2185) projected
  line L20 (16.3538, -7.9375) -> (13.8138, -7.9375) projected
  line L21 (49.911, -7.9375) -> (49.911, -10.2185) projected
  line L22 (47.371, -7.9375) -> (49.911, -7.9375) projected
  line L23 (47.371, -7.9375) -> (47.371, -10.2185) projected
  line L24 (47.371, -10.2185) -> (49.911, -10.2185) projected
  line L25 (49.911, -56.0549) -> (49.911, -12.7) projected
  line L26 (49.911, -12.7) -> (48.26, -12.7)
  line L27 (48.26, -12.7) -> (48.26, -10.2185)
  line L28 (48.26, -10.2185) -> (49.911, -10.2185)
  line L29 (49.911, -10.2185) -> (49.911, -12.7)
  line L30 (13.8138, -12.7) -> (13.8138, -56.0549) projected
  line L31 (15.4648, -49.7049) -> (15.4648, -10.2185) projected
  line L32 (13.8138, -12.7) -> (15.4648, -12.7)
  line L33 (15.4648, -12.7) -> (15.4648, -10.2185)
  line L34 (15.4648, -10.2185) -> (13.8138, -10.2185)
  line L35 (13.8138, -10.2185) -> (13.8138, -12.7)
  point P0 (0, 0)
  constraints: 24 end point, 6 parallel, 3 horizontal, 3 perpendicular
extrude "Extrusion33" add sketch "Sketch43" along normal up to surface (10.795 mm away) contours L11 L10 L9 L8 L7 L6 L5 L4 L3 L2 L1 A1 L0 A0 | L35 L18 L31 L10 | L2 L27 L24 L29 | L15 L5 L6 L7
fillet "Fillet36" radius 2.54 5 edges at (47.1212, -7.62, -62.7901) (31.8624, -7.62, -65.5799) (16.6037, -7.62, -62.7901) (13.8138, -7.62, -33.1367) (49.911, -7.62, -33.1367)
fillet "Fillet37" radius 2.54 6 edges at (49.911, -0.3175, -12.7) (49.911, -0.3175, 38.2532) (13.8138, -0.3175, 0) (13.8138, -0.3175, -12.7) (13.8138, -0.3175, 38.2532) (49.911, -0.3175, 0)
fillet "Fillet38" radius 2.54 20 edges at (49.911, -2.54, -13.97) (49.911, -2.54, -6.35) (49.911, -2.54, 1.27) (49.911, 1.905, -13.97) (49.911, 1.905, -6.35) (49.911, 1.905, 1.27) (49.911, 1.905, 36.9832) (49.911, 1.905, 44.6032) (49.911, -2.54, 36.9832) (49.911, -2.54, 44.6032) (13.8138, -2.54, 1.27) (13.8138, -2.54, -6.35) (13.8138, -2.54, -13.97) (13.8138, -2.54, 36.9832) (13.8138, -2.54, 44.6032) (13.8138, 1.905, 1.27) (13.8138, 1.905, -6.35) (13.8138, 1.905, -13.97) (13.8138, 1.905, 36.9832) (13.8138, 1.905, 44.6032)
sketch "Sketch44" plane through (49.911, -45.344, -10.2185) normal (1, 0, 0) x (0, 0, -1)
  line L0 (-61.1717, 40.264) -> (-45.9317, 40.264) projected
  line L1 (-61.1717, 40.264) -> (-61.1717, -2.281) projected
  line L2 (-61.1717, -2.281) -> (-53.081, -2.281) projected
  line L3 (-53.081, -2.281) -> (-50.8, 0) projected
  line L4 (-50.8, 0) -> (-48.519, -2.281) projected
  line L5 (-48.519, -2.281) -> (-40.381, -2.281) projected
  line L6 (-40.381, -2.281) -> (-38.1, 0) projected
  line L7 (-38.1, 0) -> (-35.819, -2.281) projected
  line L8 (-35.819, -2.281) -> (-27.681, -2.281) projected
  line L9 (-27.681, -2.281) -> (-25.4, 0) projected
  line L10 (-25.4, 0) -> (-23.119, -2.281) projected
  line L11 (-23.119, -2.281) -> (-14.981, -2.281) projected
  line L12 (-14.981, -2.281) -> (-12.7, 0) projected
  line L13 (-12.7, 0) -> (-10.419, -2.281) projected
  line L14 (-10.419, -2.281) -> (-2.281, -2.281) projected
  line L15 (-2.281, -2.281) -> (0, 0) projected
  line L16 (0, 0) -> (0, 8.138) projected
  line L17 (0, 8.138) -> (-2.281, 10.419) projected
  line L18 (-2.281, 10.419) -> (0, 12.7) projected
  line L19 (0, 12.7) -> (0, 20.838) projected
  line L20 (0, 20.838) -> (-2.281, 23.119) projected
  line L21 (-2.281, 23.119) -> (0, 25.4) projected
  line L22 (0, 25.4) -> (0, 40.264) projected
  line L23 (-12.7585, 40.264) -> (0, 40.264) projected
  line L24 (-12.7585, 49.789) -> (-12.7585, 40.264) projected
  line L25 (5.0215, 49.789) -> (-12.7585, 49.789) projected
  line L26 (5.0215, 40.264) -> (5.0215, 49.789) projected
  line L27 (45.8364, 40.264) -> (5.0215, 40.264) projected
  line L28 (45.8364, 59.949) -> (45.8364, 40.264) projected
  line L29 (45.8364, 59.949) -> (-61.1717, 59.949) projected
  line L30 (-61.1717, 49.789) -> (-61.1717, 59.949) projected
  line L31 (-45.9317, 49.789) -> (-61.1717, 49.789) projected
  line L32 (-45.9317, 40.264) -> (-45.9317, 49.789) projected
  line L33 (-27.681, 23.119) -> (-25.4, 25.4) projected
  line L34 (-25.4, 25.4) -> (-23.119, 23.119) projected
  line L35 (-23.119, 23.119) -> (-25.4, 20.838) projected
  line L36 (-25.4, 20.838) -> (-27.681, 23.119) projected
  line L37 (-40.381, 23.119) -> (-38.1, 25.4) projected
  line L38 (-38.1, 25.4) -> (-35.819, 23.119) projected
  line L39 (-35.819, 23.119) -> (-38.1, 20.838) projected
  line L40 (-38.1, 20.838) -> (-40.381, 23.119) projected
  line L41 (-53.081, 23.119) -> (-50.8, 25.4) projected
  line L42 (-50.8, 25.4) -> (-48.519, 23.119) projected
  line L43 (-48.519, 23.119) -> (-50.8, 20.838) projected
  line L44 (-50.8, 20.838) -> (-53.081, 23.119) projected
  line L45 (-12.7, 25.4) -> (-10.419, 23.119) projected
  line L46 (-10.419, 23.119) -> (-12.7, 20.838) projected
  line L47 (-12.7, 20.838) -> (-14.981, 23.119) projected
  line L48 (-14.981, 23.119) -> (-12.7, 25.4) projected
  line L49 (-53.081, 10.419) -> (-50.8, 12.7) projected
  line L50 (-50.8, 12.7) -> (-48.519, 10.419) projected
  line L51 (-48.519, 10.419) -> (-50.8, 8.138) projected
  line L52 (-50.8, 8.138) -> (-53.081, 10.419) projected
  line L53 (-27.681, 10.419) -> (-25.4, 12.7) projected
  line L54 (-25.4, 12.7) -> (-23.119, 10.419) projected
  line L55 (-23.119, 10.419) -> (-25.4, 8.138) projected
  line L56 (-25.4, 8.138) -> (-27.681, 10.419) projected
  line L57 (-40.381, 10.419) -> (-38.1, 12.7) projected
  line L58 (-38.1, 12.7) -> (-35.819, 10.419) projected
  line L59 (-35.819, 10.419) -> (-38.1, 8.138) projected
  line L60 (-38.1, 8.138) -> (-40.381, 10.419) projected
  line L61 (-14.981, 10.419) -> (-12.7, 12.7) projected
  line L62 (-12.7, 12.7) -> (-10.419, 10.419) projected
  line L63 (-10.419, 10.419) -> (-12.7, 8.138) projected
  line L64 (-12.7, 8.138) -> (-14.981, 10.419) projected
  line L65 (-54.8386, 19.0804) -> (-54.8386, 14.4576) projected
  line L66 (-54.8386, 14.4576) -> (-59.4614, 14.4576) projected
  line L67 (-59.4614, 14.4576) -> (-59.4614, 19.0804) projected
  line L68 (-59.4614, 19.0804) -> (-54.8386, 19.0804) projected
  line L69 (-42.1386, 19.0804) -> (-42.1386, 14.4576) projected
  line L70 (-42.1386, 14.4576) -> (-46.7614, 14.4576) projected
  line L71 (-46.7614, 14.4576) -> (-46.7614, 19.0804) projected
  line L72 (-46.7614, 19.0804) -> (-42.1386, 19.0804) projected
  line L73 (-16.7386, 6.3804) -> (-16.7386, 1.7576) projected
  line L74 (-16.7386, 1.7576) -> (-21.3614, 1.7576) projected
  line L75 (-21.3614, 1.7576) -> (-21.3614, 6.3804) projected
  line L76 (-21.3614, 6.3804) -> (-16.7386, 6.3804) projected
  line L77 (-34.0614, 1.7576) -> (-34.0614, 6.3804) projected
  line L78 (-34.0614, 6.3804) -> (-29.4386, 6.3804) projected
  line L79 (-29.4386, 6.3804) -> (-29.4386, 1.7576) projected
  line L80 (-29.4386, 1.7576) -> (-34.0614, 1.7576) projected
  line L81 (-16.7386, 19.0804) -> (-16.7386, 14.4576) projected
  line L82 (-16.7386, 14.4576) -> (-21.3614, 14.4576) projected
  line L83 (-21.3614, 14.4576) -> (-21.3614, 19.0804) projected
  line L84 (-21.3614, 19.0804) -> (-16.7386, 19.0804) projected
  line L85 (-4.0386, 19.0804) -> (-4.0386, 14.4576) projected
  line L86 (-4.0386, 14.4576) -> (-8.6614, 14.4576) projected
  line L87 (-8.6614, 14.4576) -> (-8.6614, 19.0804) projected
  line L88 (-8.6614, 19.0804) -> (-4.0386, 19.0804) projected
  line L89 (-29.4386, 19.0804) -> (-29.4386, 14.4576) projected
  line L90 (-29.4386, 14.4576) -> (-34.0614, 14.4576) projected
  line L91 (-34.0614, 14.4576) -> (-34.0614, 19.0804) projected
  line L92 (-34.0614, 19.0804) -> (-29.4386, 19.0804) projected
  line L93 (-8.6614, 1.7576) -> (-8.6614, 6.3804) projected
  line L94 (-8.6614, 6.3804) -> (-4.0386, 6.3804) projected
  line L95 (-4.0386, 6.3804) -> (-4.0386, 1.7576) projected
  line L96 (-4.0386, 1.7576) -> (-8.6614, 1.7576) projected
  line L97 (-46.7614, 1.7576) -> (-46.7614, 6.3804) projected
  line L98 (-46.7614, 6.3804) -> (-42.1386, 6.3804) projected
  line L99 (-42.1386, 6.3804) -> (-42.1386, 1.7576) projected
  line L100 (-42.1386, 1.7576) -> (-46.7614, 1.7576) projected
  line L101 (-59.4614, 1.7576) -> (-59.4614, 6.3804) projected
  line L102 (-59.4614, 6.3804) -> (-54.8386, 6.3804) projected
  line L103 (-54.8386, 6.3804) -> (-54.8386, 1.7576) projected
  line L104 (-54.8386, 1.7576) -> (-59.4614, 1.7576) projected
  line L105 (-21.3614, 31.7804) -> (-16.7386, 31.7804) projected
  line L106 (-16.7386, 31.7804) -> (-16.7386, 27.1576) projected
  line L107 (-16.7386, 27.1576) -> (-21.3614, 27.1576) projected
  line L108 (-21.3614, 27.1576) -> (-21.3614, 31.7804) projected
  line L109 (-46.7614, 27.1576) -> (-46.7614, 31.7804) projected
  line L110 (-46.7614, 31.7804) -> (-42.1386, 31.7804) projected
  line L111 (-42.1386, 31.7804) -> (-42.1386, 27.1576) projected
  line L112 (-42.1386, 27.1576) -> (-46.7614, 27.1576) projected
  line L113 (-34.0614, 27.1576) -> (-34.0614, 31.7804) projected
  line L114 (-34.0614, 31.7804) -> (-29.4386, 31.7804) projected
  line L115 (-29.4386, 31.7804) -> (-29.4386, 27.1576) projected
  line L116 (-29.4386, 27.1576) -> (-34.0614, 27.1576) projected
  line L117 (-4.0386, 31.7804) -> (-4.0386, 27.1576) projected
  line L118 (-4.0386, 27.1576) -> (-8.6614, 27.1576) projected
  line L119 (-8.6614, 27.1576) -> (-8.6614, 31.7804) projected
  line L120 (-8.6614, 31.7804) -> (-4.0386, 31.7804) projected
  line L121 (-59.4614, 27.1576) -> (-59.4614, 31.7804) projected
  line L122 (-59.4614, 31.7804) -> (-54.8386, 31.7804) projected
  line L123 (-54.8386, 31.7804) -> (-54.8386, 27.1576) projected
  line L124 (-54.8386, 27.1576) -> (-59.4614, 27.1576) projected
  line L125 (-40.381, -2.281) -> (-38.1, 0) projected
  line L126 (-61.1717, 40.264) -> (-61.1717, -2.281) projected
  line L127 (-59.4614, 31.7804) -> (-54.8386, 31.7804) projected
  arc A0 (-37.437, 6.03) -> (-61.1717, 33.4907) centre (-65.1903, 6.03) ccw
  line L128 (-37.437, 6.03) -> (-37.437, -0.663)
  point P0 (-10.2185, 45.344)
  constraints: 3 point on circle, 2 end point, 2 point on line, 1 centre point, 1 tangent, 1 vertical
extrude "Extrusion34" cut sketch "Sketch44" against normal through all contours A0 L57 L60 L59 L128 L7 L6 L5 L4 L3 L2 L1 | A0 L59 L60 L57
sketch "Sketch45" plane through (13.8138, -32.644, -10.2185) normal (-1, 0, 0) x (0, 0, 1)
  line L0 (42.1386, 14.4576) -> (46.7614, 14.4576) projected
  line L1 (46.7614, 14.4576) -> (46.7614, 19.0804) projected
  line L2 (46.7614, 19.0804) -> (42.1386, 19.0804) projected
  line L3 (42.1386, 19.0804) -> (42.1386, 14.4576) projected
  arc A0 (61.1717, 20.7907) -> (38.2208, -0.1208) centre (65.1903, -6.67) ccw projected
  arc A1 (37.5633, -4.0253) -> (38.2208, -0.1208) centre (65.1903, -6.67) ccw projected
  arc A2 (38.2208, -0.1208) -> (37.5633, -4.0253) centre (65.1903, -6.67) ccw
  line L4 (35.819, -2.281) -> (37.5633, -4.0253) projected
  line L5 (38.1, 0) -> (35.819, -2.281) projected
  line L6 (38.2208, -0.1208) -> (38.1, 0) projected
  line L7 (38.2208, -0.1208) -> (38.1, 0) projected
  line L8 (38.2208, -0.1208) -> (38.1, 0)
  line L9 (38.1, 0) -> (35.819, -2.281) projected
  line L10 (38.1, 0) -> (35.819, -2.281)
  line L11 (35.819, -2.281) -> (37.5633, -4.0253) projected
  line L12 (35.819, -2.281) -> (37.5633, -4.0253)
  point P0 (10.2185, 32.644)
  point P1 (38.1, -12.7)
  constraints: 6 end point, 2 perpendicular, 2 point on circle, 1 centre point, 1 coincident, 1 collinear, 1 point on line
extrude "Extrusion35" add sketch "Sketch45" against normal up to surface (2.54 mm away) contours L3 L2 L1 L0 | A2 L4 L5 L6
fillet "Fillet39" radius 8.89 1 edges at (15.0838, -11.8533, 50.9532)
mirror "Mirror4" about plane through (31.8624, 3.175, 57.15) normal (-1, 0, 0) of "Extrusion35", "Fillet39"
fillet "Fillet40" radius 0.762 8 edges at (0, -0.3175, 50.9532) (0, -0.3175, 38.2532) (0, -0.3175, 0) (0, -0.3175, -12.7) (63.7248, -0.3175, 50.9532) (63.7248, -0.3175, 38.2532) (63.5, -0.3175, 0) (63.5, -0.3175, -12.7)
equation "\"d53\" = d52"
equation "\"d65\" = d64"
equation "\"d93\" = 0.5 * d84"
equation "\"d94\" = 0.5 * d83"
body "Solid1"
